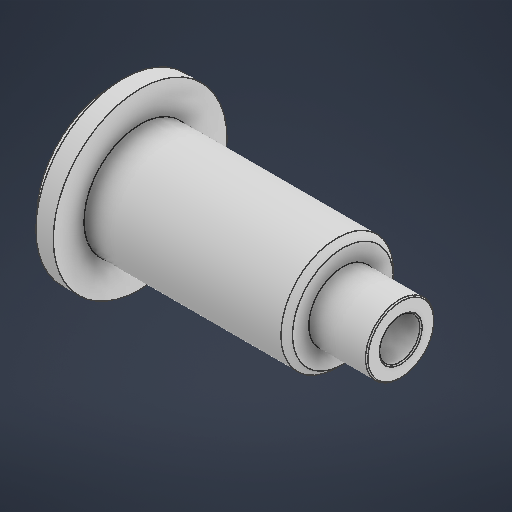
# Autodesk Inventor part: Ось односторонняя
Saved by Autodesk Inventor 2025 (Build 290162010, 162A)
## iProperties
Created: 2024-12-08
Part Number: Ось односторонняя
Material: Типовые
Document SubType Name: Modeling
Designer: Edward_Higgins
Density: 1 g/cm^3
Appearance: По умолчанию
Mass: 1.56385 g
Surface Area: 13.4378 cm^2
Volume: 1.56385 cm^3
Author: Edward_Higgins
Autodesk Inventor part; units mm, degrees
ref_plane "YZ Plane" through (0, 0, 0) normal (1, 0, 0) x (0, 1, 0)
ref_plane "XZ Plane" through (0, 0, 0) normal (0, 1, 0) x (-1, 0, 0)
ref_plane "XY Plane" through (0, 0, 0) normal (0, 0, 1) x (1, 0, 0)
sketch "Эскиз1" plane through (0, 0, 0) normal (0, 0, 1) x (1, 0, 0)
  line L0 (0, 0) -> (0, 6.4157)
  line L1 (2.5, 4.85) -> (20, 4.85)
  line L2 (20, 4.85) -> (20, 2.95)
  line L3 (20, 2.95) -> (25, 2.95)
  line L4 (25, 2.95) -> (25, 1.75)
  line L5 (25, 1.75) -> (0, 1.75)
  line L6 (0, 0) -> (17.5335, 0) construction
  line L7 (0, 6.4157) -> (1, 7.5)
  line L8 (1, 7.5) -> (2.5, 7.5)
  line L9 (2.5, 7.5) -> (2.5, 4.85)
  dimension "d0" = 5.9
  dimension "d2" = 3.5
  dimension "d3" = 9.7
  dimension "d12" = 15
  dimension "d18" = 1
  dimension "d19" = 5
  dimension "d21" = 2.5
  dimension "d22" = 17.5
  constraints: 20 end point, 6 perpendicular, 1 horizontal, 1 point on line, 1 vertical
  measures "d0" diameter of L3 L6
  measures "d2" diameter of L5 L6
  measures "d3" diameter of L1 L6
  measures "d12" diameter of L8 L6
  measures "d18" distance from line of L7.end L0
  measures "d19" distance of L2.end L3.end
  measures "d21" distance between parallel lines of L0 L9
  measures "d22" distance between parallel lines of L9 L2
revolve "Вращение1" add sketch "Эскиз1" angle 360 about axis through (0, 0, 0) along (1, 0, 0)
chamfer "Фаска1" distance 0.5 angle 45 2 edges at (20, -4.85, 0) (0, -1.75, 0)
chamfer "Фаска2" distance 0.1 angle 45 2 edges at (25, -2.95, 0) (25, -1.75, 0)
